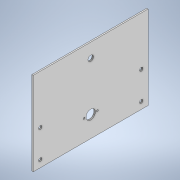
# Autodesk Inventor part: Motorblechdive
Saved by Autodesk Inventor 2022 (Build 260153000, 153)
## iProperties
Created: 2022-03-17
Part Number: Motorblechdive
Material: Generisch
Document SubType Name: Modeling
Designer: 123St
Density: 1 g/cm^3
Appearance: Vorgabe
Author: 123St
Autodesk Inventor part; units mm, degrees
ref_plane "YZ Plane" through (0, 0, 0) normal (1, 0, 0) x (0, 1, 0)
ref_plane "XZ Plane" through (0, 0, 0) normal (0, 1, 0) x (-1, 0, 0)
ref_plane "XY Plane" through (0, 0, 0) normal (0, 0, 1) x (1, 0, 0)
sketch "Skizze1" plane through (0, 0, 0) normal (1, 0, 0) x (0, 1, 0)
  line L0 (-30, 82.5) -> (30, 82.5)
  line L1 (30, 82.5) -> (30, -82.5)
  line L2 (30, -82.5) -> (-30, -82.5)
  line L3 (-30, -82.5) -> (-30, 82.5)
  line L4 (-30, 82.5) -> (30, -82.5) construction
  line L5 (30, 82.5) -> (-30, -82.5) construction
  point P0 (0, 0)
  dimension "d0" = 165
  dimension "d1" = 60
  constraints: 12 end point, 2 midpoint, 2 parallel, 1 horizontal, 1 perpendicular
  measures "d0" distance of L0.end L1.end
  measures "d1" distance of L1.end L2.end
extrude "Extrusion1" add sketch "Skizze1" along normal blind 2
sketch "Skizze2" plane through (2, 0, 0) normal (1, 0, 0) x (0, 0, -1)
  circle A0 centre (0, 0) radius 6.75
  circle A1 centre (9.5, 0) radius 1.25
  circle A2 centre (-9.5, 0) radius 1.25
  circle A3 centre (-72.5, 20) radius 2.5
  circle A4 centre (-72.5, -20) radius 2.5
  circle A5 centre (72.5, 20) radius 2.5
  circle A6 centre (72.5, -20) radius 2.5
  line L0 (-82.5, 30) -> (-82.5, -30) projected
  line L1 (-82.5, -30) -> (82.5, -30) projected
  line L2 (82.5, 30) -> (-82.5, 30) projected
  dimension "d4" = 13.5
  dimension "d5" = 19
  dimension "d6" = 9.5
  dimension "d7" = 2.5
  dimension "d8" = 2.5
  dimension "d9" = 5
  dimension "d10" = 5
  dimension "d11" = 5
  dimension "d12" = 5
  dimension "d14" = 145
  dimension "d15" = 72.5
  dimension "d16" = 145
  dimension "d17" = 72.5
  dimension "d18" = 10
  dimension "d19" = 10
  dimension "d20" = 10
  dimension "d21" = 10
  constraints: 7 centre point, 1 coincident
  measures "d4" diameter of A0
  measures "d5" distance of A2.centre A1.centre
  measures "d6" distance of point (0, 0) A1.centre
  measures "d7" diameter of A1
  measures "d8" diameter of A2
  measures "d9" diameter of A3
  measures "d10" diameter of A4
  measures "d11" diameter of A5
  measures "d12" diameter of A6
  measures "d14" distance of A3.centre A5.centre
  measures "d15" horizontal distance of point (0, 0) A5.centre
  measures "d16" distance of A6.centre A4.centre
  measures "d17" horizontal distance of A6.centre point (0, 0)
  measures "d18" distance from line of L1 A4.centre
  measures "d19" distance from line of L2 A3.centre
  measures "d20" distance from line of L2 A5.centre
  measures "d21" distance from line of L1 A6.centre
extrude "Extrusion2" cut sketch "Skizze2" against normal blind 5
sketch "Skizze3" plane through (0, 30, 82.5) normal (0, 1, 0) x (1, 0, 0)
  line L0 (0, 165) -> (0, 0) projected
  line L1 (0, 0) -> (2, 0)
  line L2 (2, 0) -> (2, 165)
  line L3 (2, 165) -> (0, 165)
  line L4 (0, 165) -> (0, 0)
  point P0 (0, 82.5)
  constraints: 8 end point, 2 parallel, 1 horizontal, 1 perpendicular
extrude "Extrusion3" add sketch "Skizze3" along normal blind 60
sketch "Skizze4" plane through (2, 0, 0) normal (1, 0, 0) x (0, 0, -1)
  circle A0 centre (0, 70) radius 4
  point P0 (0, 0)
  dimension "d26" = 70
  dimension "d27" = 8
  constraints: 1 centre point
  measures "d26" distance of point (0, 0) A0.centre
  measures "d27" diameter of A0
extrude "Extrusion4" cut sketch "Skizze4" against normal blind 45
equation "\"d6\" = 0.5 * d5"
equation "\"d15\" = 0.5 * d14"
equation "\"d17\" = 0.5 * d16"
equation "\"d22\" = d11"
